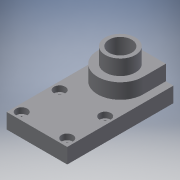
# Autodesk Inventor part: Holes
Saved by Autodesk Inventor 2017 (Build 210142000, 142)
## iProperties
Created: 2013-12-04
Part Number: Holes
Material: Generic
Document SubType Name: Modeling
Designer: John
Density: 1 g/cm^3
Appearance: Default
Author: John
Autodesk Inventor part; units mm, degrees
ref_plane "YZ Plane" through (0, 0, 0) normal (1, 0, 0) x (0, 1, 0)
ref_plane "XZ Plane" through (0, 0, 0) normal (0, 1, 0) x (-1, 0, 0)
ref_plane "XY Plane" through (0, 0, 0) normal (0, 0, 1) x (1, 0, 0)
sketch "Sketch1" plane through (0, 0, 0) normal (0, 1, 0) x (-1, 0, 0)
  line L0 (0, 0) -> (-50.8, 0)
  line L1 (-50.8, 0) -> (-50.8, -88.9)
  line L2 (-50.8, -88.9) -> (0, -88.9)
  line L3 (0, -88.9) -> (0, 0)
  dimension "d0" = 50.8
  dimension "d1" = 88.9
  constraints: 8 end point, 2 parallel, 1 horizontal, 1 perpendicular
  measures "d0" distance of L2.end L1.end
  measures "d1" distance of L1.end L0.end
extrude "Extrusion1" add sketch "Sketch1" along normal blind 12.7
sketch "Sketch2" plane through (0, 12.7, 0) normal (0, 1, 0) x (1, 0, 0)
  line L0 (50.8, 0) -> (50.8, 88.9) projected
  line L1 (50.8, 88.9) -> (0, 88.9) projected
  line L2 (0, 88.9) -> (0, 0) projected
  line L3 (6.35, 88.9) -> (44.45, 88.9)
  line L4 (44.45, 88.9) -> (44.45, 69.85)
  line L5 (44.45, 69.85) -> (6.35, 69.85)
  line L6 (6.35, 69.85) -> (6.35, 88.9)
  line L7 (6.35, 79.375) -> (0, 79.375) construction
  line L8 (44.45, 79.375) -> (50.8, 79.375) construction
  circle A0 centre (25.4, 69.85) radius 19.05
  dimension "d4" = 19.05
  dimension "d5" = 6.35
  constraints: 12 end point, 3 midpoint, 3 perpendicular, 3 point on line, 2 parallel, 1 collinear, 1 horizontal, 1 horizontal alignment, 2 other
  measures "d4" distance of L3.end L4.end
  measures "d5" distance between parallel lines of L2 L6
extrude "Extrusion2" add sketch "Sketch2" along normal blind 12.7
sketch "Sketch3" plane through (0, 25.4, 0) normal (0, 1, 0) x (1, 0, 0)
  arc A0 (6.35, 69.85) -> (44.45, 69.85) centre (25.4, 69.85) ccw projected
  circle A1 centre (25.4, 69.85) radius 12.7
  point P0 (0, 0)
  dimension "d8" = 25.4
  constraints: 1 centre point, 1 coincident
  measures "d8" diameter of A1
extrude "Extrusion3" add sketch "Sketch3" along normal blind 12.7
sketch "Sketch6" plane through (0, 12.7, 0) normal (0, 1, 0) x (1, 0, 0)
  line L0 (0, 88.9) -> (0, 0) projected
  line L1 (0, 0) -> (50.8, 0) projected
  line L2 (50.8, 0) -> (50.8, 88.9) projected
  line L3 (44.45, 88.9) -> (44.45, 6.35) construction
  line L4 (44.45, 6.35) -> (6.35, 6.35) construction
  line L5 (6.35, 6.35) -> (6.35, 88.9) construction
  line L6 (6.35, 38.1) -> (44.45, 38.1) construction
  dimension "d35" = 6.35
  dimension "d36" = 31.75
  constraints: 8 end point, 2 point on line, 1 perpendicular, 2 other
  measures "d35" distance between parallel lines of L1 L4
  measures "d36" distance between parallel lines of L4 L6
hole "Hole3" at (25.4, 38.1, -69.85) direction (0, -1, 0) diameter 19.05 end through all
hole "Hole4" at (6.35, 12.7, -6.35) at (6.35, 12.7, -38.1) at (44.45, 12.7, -6.35) at (44.45, 12.7, -38.1) direction (0, -1, 0) diameter 5.1054 end through all counterbore diameter 9.525 counterbore depth 4.826 clearance for "Socket Head Cap Screw" size "#10" standard "Ansi Unified Screw Threads"
body "Solid1"
